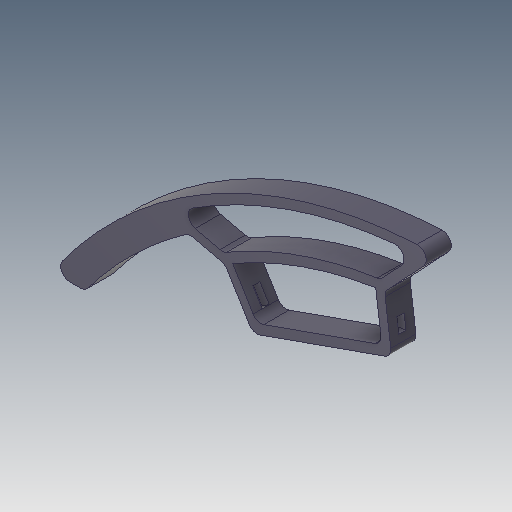
# Autodesk Inventor part: Bumper
Saved by Autodesk Inventor 2017 (Build 210142000, 142)
## iProperties
Created: 2017-05-08
Part Number: Bumper
Material: ABS Plastic
Document SubType Name: Modeling
Designer: zallen
Density: 1.06 g/cm^3
Appearance: Default Plastic
Mass: 72.8492 g
Surface Area: 267.673 cm^2
Volume: 68.7257 cm^3
Author: zallen
Autodesk Inventor part; units mm, degrees
ref_plane "YZ Plane" through (0, 0, 0) normal (1, 0, 0) x (0, 1, 0)
ref_plane "XZ Plane" through (0, 0, 0) normal (0, 1, 0) x (-1, 0, 0)
ref_plane "XY Plane" through (0, 0, 0) normal (0, 0, 1) x (1, 0, 0)
sketch "Sketch1" plane through (0, 0, 0) normal (0, 0, 1) x (1, 0, 0)
  circle A0 centre (0, -228.6) radius 228.6 construction
  line L0 (0, 0) -> (0, 15) construction
  line L1 (0, 15) -> (-3, 15) construction
  line L2 (0, 0) -> (-100, 0) construction
  line L3 (0, 0) -> (0, -85) construction
  line L4 (0, 15) -> (0, 30) construction
  line L5 (0, -85) -> (-177.8679, -85) construction
  line L6 (-177.8679, -85) -> (-196.774, -85) construction
  circle A1 centre (0, -228.6) radius 243.6 construction
  circle A2 centre (0, -228.6) radius 258.6 construction
  arc A3 (0, 30) -> (-215.0651, -85) centre (0, -228.6) ccw
  line L7 (-30, -1.9771) -> (0, 30)
  line L8 (-118.8814, -33.3433) -> (-139.0909, -28.6133)
  line L9 (-196.774, -85) -> (-215.0651, -85) construction
  line L10 (-215.0651, -85) -> (-196.774, -85)
  arc A4 (-139.0909, -28.6133) -> (-196.774, -85) centre (0, -228.6) ccw
  circle A5 centre (0, -228.6) radius 233.6 construction
  circle A6 centre (0, -228.6) radius 253.6 construction
  line L11 (-119.7215, -28.0115) -> (-146.6573, -21.7073)
  line L12 (-32.4328, 2.7376) -> (-11.8047, 24.7251)
  arc A7 (-32.4328, 2.7376) -> (-119.7215, -28.0115) centre (0, -228.6) ccw
  arc A8 (-11.8047, 24.7251) -> (-146.6573, -21.7073) centre (0, -228.6) ccw
  line L13 (-118.8814, -33.3433) -> (0, -228.6) construction
  line L14 (-30, -1.9771) -> (0, -228.6) construction
  line L15 (-118.8814, -33.3433) -> (-103.2801, -58.9675)
  line L16 (-30, -1.9771) -> (-26.063, -31.7176)
  line L17 (-103.2801, -58.9675) -> (-26.063, -31.7176)
  line L18 (-114.6107, -30.7431) -> (-101.1189, -52.9026)
  line L19 (-101.1189, -52.9026) -> (-31.5521, -28.3525)
  line L20 (-31.5521, -28.3525) -> (-34.9568, -2.6332)
  arc A9 (-34.9568, -2.6332) -> (-114.6107, -30.7431) centre (0, -228.6) ccw
  dimension "d2" = 457.2
  dimension "d3" = 228.6
  dimension "d6" = 3
  dimension "d7" = 100
  dimension "d9" = 85
  dimension "d13" = 15
  dimension "d14" = 15
  dimension "d18" = 30
  dimension "d21" = 120
  dimension "d22" = 20.2095
  dimension "d23" = 467.2
  dimension "d24" = 507.2
  dimension "d25" = 5
  dimension "d26" = 5
  dimension "d27" = 30
  dimension "d28" = 30
  dimension "d29" = 5
  dimension "d30" = 228.6547
  constraints: 42 end point, 22 point on circle, 10 centre point, 6 concentric, 5 horizontal, 3 coincident, 3 vertical, 2 parallel, 2 point on line, 1 tangent, 2 other
  measures "d2" diameter of A0
  measures "d3" distance of A0.centre L0.start
  measures "d6" distance of L0.end L1.end
  measures "d7" distance of L0.start L2.end
  measures "d9" distance of L0.start L3.end
  measures "d13" distance of L0.start L0.end
  measures "d14" distance of L0.end L4.end
  measures "d18" distance from line of L7.start L3
  measures "d21" angle of L7 L8
  measures "d22" horizontal distance of L8.start L8.end
  measures "d23" diameter of A5
  measures "d24" diameter of A6
  measures "d25" distance between parallel lines of L7 L12
  measures "d26" distance between parallel lines of L8 L11
  measures "d27" distance of L8.start L15.end
  measures "d28" distance of L7.start L16.end
  measures "d29" distance between parallel lines of L15 L18
  measures "d30" radius of A9
extrude "Extrusion1" add sketch "Sketch1" along normal blind 14
fillet "Fillet1" radius 5 14 edges at (-30, -1.9771, 7) (-118.8814, -33.3433, 7) (-139.0909, -28.6133, 7) (-11.8047, 24.7251, 7) (-146.6573, -21.7073, 7) (0, 30, 7) (-32.4328, 2.7376, 7) (-101.1189, -52.9026, 7) (-31.5521, -28.3525, 7) (-119.7215, -28.0115, 7) (-196.774, -85, 7) (-215.0651, -85, 7) (-26.063, -31.7176, 7) (-103.2801, -58.9675, 7)
sketch "Sketch2" plane through (-26.5953, -27.6963, 14) normal (0.9913515, 0.1312336, 0) x (0, 0, -1)
  line L0 (5, 4.0564) -> (9, 4.0564)
  line L1 (9, 4.0564) -> (9, 12.0564)
  line L2 (9, 12.0564) -> (5, 12.0564)
  line L3 (5, 12.0564) -> (5, 4.0564)
  line L4 (14, 0) -> (14, 23.5741) projected
  line L5 (0, 0) -> (0, 23.5741) projected
  line L6 (5, 12.0564) -> (9, 12.0564)
  line L7 (5, 4.0564) -> (9, 4.0564)
  line L8 (0, 4.0564) -> (14, 4.0564) projected
  point P0 (14, 23.9666)
  dimension "d34" = 5
  dimension "d35" = 5
  dimension "d46" = 8
  constraints: 12 end point, 3 equal length, 1 horizontal, 1 perpendicular, 1 point on line
  measures "d34" distance between parallel lines of L4 L1
  measures "d35" distance between parallel lines of L5 L3
  measures "d46" distance between parallel lines of L2 L0
extrude "Extrusion2" cut sketch "Sketch2" against normal blind 5
sketch "Sketch3" plane through (-105.3896, -55.5028, 0) normal (-0.8541413, -0.5200409, 0) x (0, 0, 1)
  line L0 (9, 14.0564) -> (9, 4.0564)
  line L1 (9, 4.0564) -> (5, 4.0564)
  line L2 (0, 4.0564) -> (14, 4.0564) projected
  line L3 (5, 14.0564) -> (9, 14.0564)
  line L4 (14, 4.0564) -> (14, 25.9436) projected
  line L5 (5, 4.0564) -> (5, 14.0564)
  line L6 (0, 25.9436) -> (0, 4.0564) projected
  point P0 (0, -7.3997)
  dimension "d38" = 5
  dimension "d39" = 5
  dimension "d40" = 10
  dimension "d41" = 10
  dimension "d42" = 90
  constraints: 8 end point, 2 vertical, 1 point on line
  measures "d38" distance between parallel lines of L4 L0
  measures "d39" distance between parallel lines of L6 L5
  measures "d40" distance of L0.start L0.end
  measures "d41" distance of L1.end L3.start
  measures "d42" angle of L5 L1
extrude "Extrusion3" cut sketch "Sketch3" against normal blind 5
body "Solid1"
